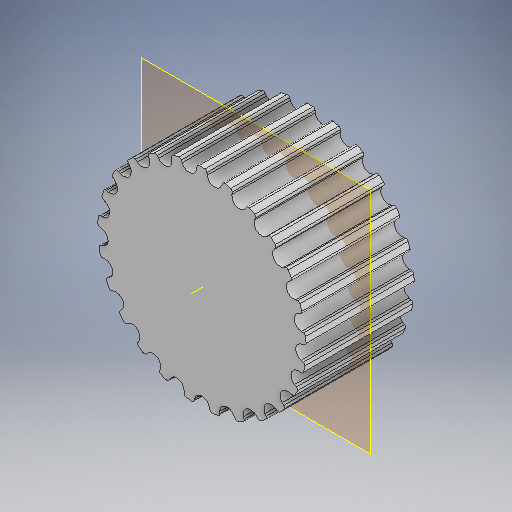
# Autodesk Inventor part: Small_Pulley
Saved by Autodesk Inventor 2025.2 (Build 292293000, 293)
## iProperties
Created: 2025-04-06
Part Number: Small_Pulley
Material: Generic
Document SubType Name: Modeling
Designer: Tiago
Density: 1 g/cm^3
Appearance: Default
Author: Tiago
Autodesk Inventor part; units mm, degrees
ref_plane "YZ Plane" through (0, 0, 0) normal (1, 0, 0) x (0, 1, 0)
ref_plane "XZ Plane" through (0, 0, 0) normal (0, 1, 0) x (-1, 0, 0)
sketch "Sketch1" plane through (0, 0, 0) normal (0, 0, 1) x (1, 0, 0)
  circle A0 centre (0, 0) radius 7.9577
  dimension "np" = 15.9155
  constraints: 1 centre point, 1 coincident
  measures "np" diameter of A0
extrude "Extrusion1" add sketch "Sketch1" along normal mid plane 8
sketch "Sketch2" plane through (0, 0, 4) normal (0, 0, 1) x (1, 0, 0)
  line L0 (0, 0) -> (0, 9.7627) construction
  circle A0 centre (0, 0) radius 7.9577 construction
  line L1 (0, 7.9577) -> (0, 7.7077)
  circle A1 centre (0, 0) radius 7.9577 construction
  line L2 (0, 0) -> (0.9974, 7.895) construction
  line L3 (0.9974, 7.895) -> (0.941, 7.4485) construction
  arc A2 (0.22, 7.7046) -> (0, 7.7077) centre (0, 0) ccw
  line L4 (0.22, 7.7046) -> (0.22, 7.5546) construction
  arc A3 (0.37, 7.5546) -> (0.22, 7.7046) centre (0.22, 7.5546) ccw
  line L5 (0.9974, 7.895) -> (1.3928, 7.8349) construction
  line L6 (1.3928, 7.8349) -> (1.3598, 7.6174) construction
  line L7 (0.22, 7.5546) -> (0.37, 7.5546) construction
  arc A4 (0.3691, 7.5711) -> (0.3938, 7.3924) centre (1.3598, 7.6174) ccw
  arc A5 (0.3938, 7.3924) -> (1.4569, 7.2581) centre (0.941, 7.4485) ccw
  arc A6 (1.3214, 7.8458) -> (1.3195, 7.8476) centre (0.941, 7.4485) ccw
  line L8 (1.979, 7.7077) -> (1.9168, 7.4656)
  arc A7 (1.9168, 7.4656) -> (1.703, 7.5173) centre (0, 0) ccw
  line L9 (1.703, 7.5173) -> (1.6657, 7.372) construction
  arc A8 (1.703, 7.5173) -> (1.5204, 7.4093) centre (1.6657, 7.372) ccw
  line L10 (0.9974, 7.895) -> (0.5994, 7.9351) construction
  line L11 (0.5994, 7.9351) -> (0.5773, 7.7163) construction
  arc A9 (1.4569, 7.2581) -> (1.5254, 7.425) centre (0.5773, 7.7163) ccw
  arc A10 (0.3938, 7.3924) -> (1.4569, 7.2581) centre (0.941, 7.4485) ccw
  arc A11 (1.979, 7.7077) -> (0, 7.9577) centre (0, 0) ccw
  point P0 (1.3837, 7.7749)
  point P1 (0.5933, 7.8747)
  point P2 (0.37, 7.5546)
  point P3 (1.5204, 7.4093)
  dimension "d3" = 0.25
  dimension "d29" = 7.2
  dimension "d30" = 0.45
  dimension "d38" = 0.22
  dimension "d39" = 0.15
  dimension "d49" = 0.4
  dimension "d50" = 0.22
  constraints: 25 point on circle, 24 end point, 12 symmetric about line, 10 centre point, 6 coincident, 6 point on line, 2 vertical, 1 horizontal, 1 perpendicular, 1 vertical alignment, 5 other
  measures "d3" distance of L1.start L1.end
  measures "d29" angle of L0 L2
  measures "d30" distance of L2.end L3.end
  measures "d39" distance of L4.start L4.end
  measures "d49" distance of L2.end L5.end
  measures "d50" distance of L5.end L6.end
extrude "Extrusion3" cut sketch "Sketch2" against normal up to surface (8 mm away) contours A11 A6 A4 A3 A2 L1 | A11 A6 A5 | A11 L8 A7 A8 A9 A6
pattern_circular "Circular Pattern2" count 25 over 360 about axis through (0, 0, -10) along (0, 0, 1) of "Extrusion3"
equation "\"p\" = 2"
body "Solid1"
